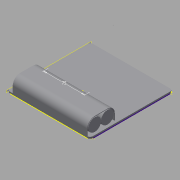
# Autodesk Inventor part: Part1
Saved by Autodesk Inventor 2015 (Build 190159000, 159)
## iProperties
Created: 2015-11-04
Part Number: Part1
Material: Generic
Document SubType Name: Modeling
Designer: Ross
Density: 1 g/cm^3
Appearance: Default
Author: Ross
Autodesk Inventor part; units mm, degrees
sketch "Sketch1" plane through (0, 0, 0) normal (0, 1, 0) x (-1, 0, 0)
  line L0 (0, 0) -> (75, 0)
  line L1 (0, 0) -> (-75, 0)
  line L2 (75, 0) -> (75, 75)
  line L3 (75, 75) -> (-75, 75)
  line L4 (-75, 75) -> (-75, 0)
  line L5 (-75, 0) -> (-75, -75)
  line L6 (-75, -75) -> (75, -75)
  line L7 (75, -69.5548) -> (75, 0)
  line L8 (75, -75) -> (75, -69.5548)
  line L9 (-75, 75) -> (-75, 65)
  dimension "d4" = 10
  constraints: 20 end point, 5 perpendicular, 4 point on line, 2 horizontal, 1 vertical
  measures "d4" distance of L3.end L9.end
extrude "Extrusion1" add sketch "Sketch1" along normal blind 3
ref_plane "Work Plane1" through (75, 0, 0) normal (1, 0, 0) x (0, 1, 0)
sketch "Sketch3" plane through (75, 0, 0) normal (1, 0, 0) x (0, 1, 0)
  line L0 (3, 75) -> (3, 65)
  line L1 (3, 75) -> (3, -75) projected
  line L2 (3, 65) -> (3, 53.5)
  line L3 (3, 53.5) -> (14.5, 53.5)
  circle A0 centre (14.5, 53.5) radius 11.5
  line L4 (3, 53.5) -> (3, 30.5)
  line L5 (3, 30.5) -> (14.5, 30.5)
  circle A1 centre (14.5, 30.5) radius 11.5
  point P0 (0, 0)
  dimension "d12" = 10
  dimension "d13" = 11.5
  dimension "d14" = 11.5
  dimension "d15" = 23
  constraints: 10 end point, 3 point on line, 2 coincident, 2 horizontal alignment, 2 perpendicular, 4 other
  measures "d12" distance of L0.start L0.end
  measures "d13" distance of L0.end L2.end
  measures "d14" distance of L2.end L3.end
  measures "d15" distance of L2.end L4.end
extrude "Extrusion2" add sketch "Sketch3" against normal blind 135 contours A0 | A1
sketch "Sketch4" plane through (0, 3, 0) normal (0, 1, 0) x (1, 0, 0)
  point P0 (0, 0)
sketch "Sketch5" plane through (0, 3, 0) normal (0, 1, 0) x (1, 0, 0)
  point P0 (0, 0)
sketch "Sketch6" plane through (75, 0, 0) normal (1, 0, 0) x (0, 1, 0)
  arc A0 (14.5, 42) -> (3, 53.5) centre (14.5, 53.5) ccw projected
  line L0 (3, 75) -> (3, 53.5) projected
  arc A1 (3, 30.5) -> (14.5, 42) centre (14.5, 30.5) ccw projected
  line L1 (3, 30.5) -> (3, -75) projected
  line L2 (14.5, 66) -> (3, 66)
  line L3 (14.5, 18) -> (3, 18)
  arc A2 (27, 53.5) -> (14.5, 66) centre (14.5, 53.5) ccw
  line L4 (27, 53.5) -> (27, 30.5)
  arc A3 (14.5, 18) -> (27, 30.5) centre (14.5, 30.5) ccw
  line L5 (3, 66) -> (3, 67)
  line L6 (3, 67) -> (14.5, 67)
  arc A4 (28, 53.5) -> (14.5, 67) centre (14.5, 53.5) ccw
  line L7 (28, 53.5) -> (28, 30.5)
  arc A5 (14.5, 17) -> (28, 30.5) centre (14.5, 30.5) ccw
  line L8 (14.5, 17) -> (3, 17)
  line L9 (3, 67) -> (3, 66)
  line L10 (3, 18) -> (3, 17)
  point P0 (0, 0)
  dimension "d20" = 12.5
  dimension "d21" = 1
  constraints: 18 end point, 8 point on circle, 4 centre point, 4 coincident, 4 perpendicular, 4 point on line, 3 vertical, 1 collinear
  measures "d20" distance of L2.start A0.centre
  measures "d21" distance of L2.end L5.end
extrude "Extrusion3" add sketch "Sketch6" against normal blind 135 contours L0 L6 A4 L7 A5 L8 L1 L3 A3 L4 A2 L2
ref_plane "Work Plane2" through (-75, 0, 75) normal (0, 0, 1) x (1, 0, 0)
sketch "Sketch8" plane through (-75, 0, 75) normal (0, 0, 1) x (1, 0, 0)
  line L0 (0, 3) -> (150, 3)
  line L1 (150, 3) -> (150, 0)
  line L2 (150, 0) -> (0, 0)
  line L3 (0, 0) -> (0, 3)
  point P0 (75, 0)
  constraints: 8 end point, 2 parallel, 1 horizontal, 1 perpendicular
extrude "Extrusion5" cut sketch "Sketch8" against normal blind 8
ref_plane "Work Plane3" through (-75, 0, -75) normal (-1, 0, 0) x (0, 0, 1)
sketch "Sketch9" plane through (-75, 0, -75) normal (-1, 0, 0) x (0, 0, 1)
  line L0 (0, 3.2367) -> (142, 3.2367)
  line L1 (142, 3.2367) -> (142, 0)
  line L2 (142, 0) -> (0, 0)
  line L3 (0, 0) -> (0, 3.2367)
  point P0 (75, 0)
  constraints: 8 end point, 2 parallel, 1 horizontal, 1 perpendicular
extrude "Extrusion6" cut sketch "Sketch9" against normal blind 5
sketch "Sketch10" plane through (75, 0, 0) normal (1, 0, 0) x (0, 1, 0)
  line L0 (3, 67) -> (0, 67)
  line L1 (0, 67) -> (0, -82.8799)
  line L2 (0, -82.8799) -> (3, -82.8799)
  line L3 (3, -82.8799) -> (3, 67)
  point P0 (0, 0)
  constraints: 8 end point, 2 parallel, 1 horizontal, 1 perpendicular
extrude "Extrusion7" add sketch "Sketch10" along normal blind 5
ref_plane "Work Plane4" through (75, 0, 0) normal (-1, 0, 0) x (0, 0, 1)
sketch "Sketch11" plane through (75, 0, 0) normal (-1, 0, 0) x (0, 0, 1)
  line L0 (-75, 3) -> (-82.8799, 3)
  line L1 (-82.8799, 3) -> (-82.8799, 0)
  line L2 (-82.8799, 0) -> (-75, 0)
  line L3 (-75, 0) -> (-75, 3)
  point P0 (0, 0)
  constraints: 8 end point, 2 parallel, 1 horizontal, 1 perpendicular
extrude "Extrusion8" cut sketch "Sketch11" against normal blind 5
sketch "Sketch12" plane through (80, 3, -75) normal (0, 0, -1) x (-1, 0, 0)
  line L0 (0, 0) -> (150, 0)
  line L1 (150, 0) -> (150, -3)
  line L2 (150, -3) -> (0, -3)
  line L3 (0, -3) -> (0, 0)
  point P0 (80, -3)
  constraints: 8 end point, 2 parallel, 1 horizontal, 1 perpendicular
extrude "Extrusion9" add sketch "Sketch12" along normal blind 8
fillet "Fillet1" radius 5 1 edges at (80, 1.5, 67)
fillet "Fillet2" radius 5 1 edges at (80, 1.5, -83)
fillet "Fillet3" radius 5 1 edges at (-70, 1.5, 67)
fillet "Fillet4" radius 5 1 edges at (-70, 1.5, -83)
sketch "Sketch13" plane through (0, 0, 0) normal (0, -1, 0) x (1, 0, 0)
  line L0 (80, 62) -> (80, -78)
  arc A0 (75, -83) -> (80, -78) centre (75, -78) ccw projected
  line L1 (80, -78) -> (80, -8)
  line L2 (80, -8) -> (-70, -8)
  line L3 (-70, 62) -> (-70, -78) projected
  line L4 (-70, -8) -> (-70, -78)
  line L5 (-70, -78) -> (-70, -8)
  line L6 (-70, 62) -> (-70, -8)
  line L7 (-70, -8) -> (5, -8)
  line L8 (5, -8) -> (5, 67)
  line L9 (75, 67) -> (-65, 67) projected
  line L10 (5, -8) -> (5, -83)
  point P0 (0, 0)
  dimension "d47" = 75
  constraints: 18 end point, 4 midpoint, 3 collinear, 1 point on line, 1 tangent, 1 vertical
  measures "d47" distance of L2.end L7.end
ref_plane "Work Plane5" through (-70, 0, -75) normal (-1, 0, 0) x (0, 0, 1)
sketch "Sketch14" plane through (-70, 0, -75) normal (-1, 0, 0) x (0, 0, 1)
  line L0 (137, 3) -> (-3, 3) projected
  line L1 (137, 0) -> (-3, 0) projected
  line L2 (67, 0) -> (67, 3)
  arc A0 (74.2639, 3) -> (75, 3) centre (74.6319, 3) ccw
  line L3 (67, 0) -> (59.35, 0)
  line L4 (67, 0) -> (74.65, 0)
  line L5 (74.65, 0) -> (74.65, -17)
  arc A1 (59.35, -17) -> (74.65, -17) centre (67, -10) ccw
  line L6 (74.65, -17) -> (74.65, 0)
  line L7 (59.35, -17) -> (59.35, 0)
  line L8 (59.35, 0) -> (74.65, 0)
  line L9 (74.65, -17) -> (74.65, 0)
  line L10 (59.1282, 0) -> (57.1283, 0)
  line L11 (59.35, 0) -> (57.35, 0)
  line L12 (57.35, -17) -> (59.35, -17)
  line L13 (74.65, 0) -> (76.65, 0)
  line L14 (76.65, -17) -> (74.65, -17)
  arc A2 (57.35, -17) -> (76.65, -17) centre (67, -10) ccw
  line L15 (74.65, 0) -> (74.65, -17)
  line L16 (76.65, 0) -> (85.15, 0)
  arc A3 (85.15, 0) -> (76.65, -8.5) centre (86.1766, -9.5266) ccw
  arc A4 (57.35, -8.5) -> (48.85, 0) centre (47.8234, -9.5266) ccw
  line L17 (57.35, -8.5) -> (57.35, -17)
  line L18 (76.65, -17) -> (76.65, -8.5)
  line L19 (48.85, 0) -> (59.35, 0)
  line L20 (74.65, 0) -> (85.15, 0)
  line L21 (74.65, 0) -> (74.65, -17)
  point P0 (75, 0)
  dimension "d49" = 7.65
  dimension "d50" = 7.65
  dimension "d52" = 17
  dimension "d53" = 2
  dimension "d54" = 2
  dimension "d55" = 8.5
  constraints: 40 end point, 11 point on circle, 5 centre point, 4 collinear, 3 perpendicular, 3 point on line, 3 symmetric about line, 1 coincident, 1 horizontal, 1 midpoint, 1 vertical, 9 other
  measures "d49" distance of L2.start L3.end
  measures "d50" distance of L2.start L4.end
  measures "d52" distance of L4.end L5.end
  measures "d53" distance of L3.end L11.end
  measures "d54" distance of L4.end L13.end
  measures "d55" distance of L13.end L16.end
extrude "Extrusion10" add sketch "Sketch14" against normal blind 18 contours A3 L18 L14 L5 L1 | A2 L12 A1 L14 | L17 A4 L1 L7 L12
body "Solid1"
